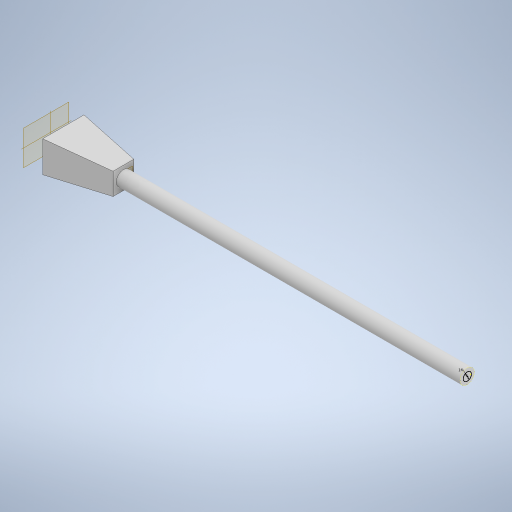
# Autodesk Inventor part: Friend_gun_collision
Saved by Autodesk Inventor 2024 (Build 280153000, 153)
## iProperties
Created: 2026-05-24
Part Number: Friend_gun_collision
Material: Generic
Document SubType Name: Modeling
Designer: warny
Density: 1 g/cm^3
Appearance: Default
Author: warny
Autodesk Inventor part; units mm, degrees
ref_plane "XZ Plane" through (0, 0, 0) normal (0, 1, 0) x (-1, 0, 0)
ref_plane "XY Plane" through (0, 0, 0) normal (0, 0, 1) x (1, 0, 0)
ref_plane "Work Plane1" through (29.8, 0, 0) normal (1, 0, 0) x (0, 1, 0)
sketch "Sketch1" plane through (29.8, 0, 0) normal (1, 0, 0) x (0, 1, 0)
  line L0 (-27, 43.9) -> (27, 43.9)
  line L1 (27, 43.9) -> (27, -27.7)
  line L2 (27, -27.7) -> (-27, -27.7)
  line L3 (-27, -27.7) -> (-27, 43.9)
  line L4 (0, -42.02) -> (0, 58.22) projected
  line L5 (-37.8, 0) -> (37.8, 0) projected
  point P0 (0, 0)
  dimension "d1" = 27
  dimension "d2" = 27
  dimension "d3" = 43.9
  dimension "d4" = 27.7
  constraints: 8 end point, 2 parallel, 1 horizontal, 1 perpendicular
  measures "d1" distance between parallel lines of L3 L4
  measures "d2" distance between parallel lines of L4 L1
  measures "d3" distance between parallel lines of L5 L0
  measures "d4" distance between parallel lines of L5 L2
ref_plane "Work Plane2" through (131.6, 0, 0) normal (1, 0, 0) x (0, 1, 0)
sketch "Sketch2" plane through (131.6, 0, 0) normal (1, 0, 0) x (0, 1, 0)
  line L0 (-19, 23.7) -> (19, 23.7)
  line L1 (19, 23.7) -> (19, -12.3)
  line L2 (19, -12.3) -> (-19, -12.3)
  line L3 (-19, -12.3) -> (-19, 23.7)
  line L4 (-26.6, 0) -> (26.6, 0) projected
  line L5 (0, -19.5) -> (0, 30.9) projected
  point P0 (0, 0)
  dimension "d6" = 23.7
  dimension "d7" = 12.3
  dimension "d8" = 19
  dimension "d9" = 19
  constraints: 8 end point, 2 parallel, 1 horizontal, 1 perpendicular
  measures "d6" distance between parallel lines of L0 L4
  measures "d7" distance between parallel lines of L4 L2
  measures "d8" distance between parallel lines of L3 L5
  measures "d9" distance between parallel lines of L5 L1
loft "Loft1" add profiles "Sketch2", "Sketch1"
sketch "Sketch3" plane through (131.6, 0, 0) normal (1, 0, 0) x (0, 1, 0)
  line L0 (0, -19.5) -> (0, 30.9) projected
  circle A0 centre (0, 5.7) radius 12.5
  point P0 (0, 0)
  dimension "d14" = 5.7
  dimension "d15" = 25
  constraints: 1 centre point, 1 coincident, 1 midpoint
  measures "d14" distance of point (0, 0) point (0, 5.7)
  measures "d15" diameter of A0
extrude "Extrusion1" add sketch "Sketch3" along normal blind 596.1
sketch "Sketch5" plane through (727.7, 0, 5.7) normal (1, 0, 0) x (0, 0, -1)
  circle A0 centre (0, 0) radius 12.5 construction
  circle A1 centre (0, 0) radius 7
  point P0 (5.7, 0)
  dimension "d19" = 14
  constraints: 1 centre point, 1 coincident
  measures "d19" diameter of A1
body "Solid1"
